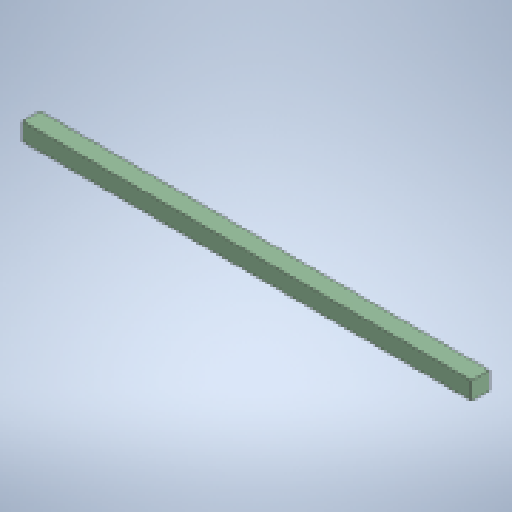
# Autodesk Inventor part: 7'5x4x4
Saved by Autodesk Inventor 2025.1 (Build 291241020, 241B)
## iProperties
Created: 2024-09-16
Part Number: 7'5x4x4
Material: Generic
Document SubType Name: Modeling
Designer: User
Density: 1 g/cm^3
Appearance: Default
Author: User
Autodesk Inventor part; units mm, degrees
ref_plane "YZ Plane" through (0, 0, 0) normal (1, 0, 0) x (0, 1, 0)
ref_plane "XZ Plane" through (0, 0, 0) normal (0, 1, 0) x (-1, 0, 0)
ref_plane "XY Plane" through (0, 0, 0) normal (0, 0, 1) x (1, 0, 0)
sketch "Sketch1" plane through (0, 0, 0) normal (1, 0, 0) x (0, 1, 0)
  line L0 (-44.45, -44.45) -> (44.45, -44.45)
  line L1 (44.45, -44.45) -> (44.45, 44.45)
  line L2 (44.45, 44.45) -> (-44.45, 44.45)
  line L3 (-44.45, 44.45) -> (-44.45, -44.45)
  line L4 (-44.45, -44.45) -> (44.45, 44.45) construction
  line L5 (44.45, -44.45) -> (-44.45, 44.45) construction
  point P0 (0, 0)
  dimension "d0" = 88.9
  dimension "d1" = 88.9
  constraints: 12 end point, 2 midpoint, 2 parallel, 1 horizontal, 1 perpendicular
  measures "d0" distance of L0.end L1.end
  measures "d1" distance of L1.end L2.end
extrude "Extrusion1" add sketch "Sketch1" along normal mid plane 2260.6
body "Solid1"
